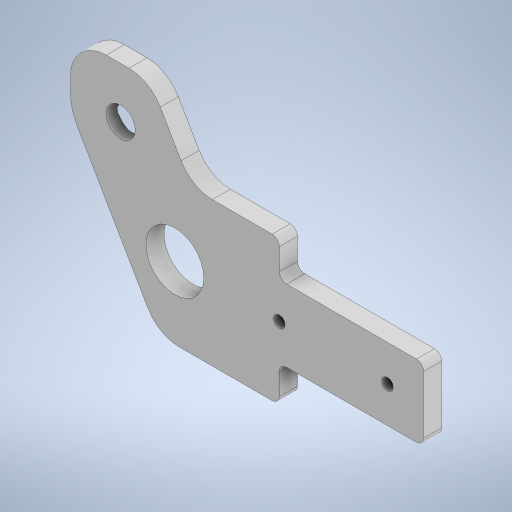
# Autodesk Inventor part: RP_Calf-Link-cover-Inside-Right
Saved by Autodesk Inventor 2024.3 (Build 283343000, 343)
## iProperties
Created: 2025-04-12
Part Number: RP_Calf-Link-cover-Inside-Right
Material: 一般
Document SubType Name: Modeling
Designer: 佐藤智貴
Density: 1 g/cm^3
Appearance: 既定
Author: 佐藤智貴
Autodesk Inventor part; units mm, degrees
ref_plane "YZ Plane" through (0, 0, 0) normal (1, 0, 0) x (0, 1, 0)
ref_plane "XZ Plane" through (0, 0, 0) normal (0, 1, 0) x (-1, 0, 0)
ref_plane "XY Plane" through (0, 0, 0) normal (0, 0, 1) x (1, 0, 0)
sketch "スケッチ1" plane through (0, 0, 0) normal (0, 0, 1) x (1, 0, 0)
  line L0 (0, 0) -> (98, 0)
  line L1 (98, 0) -> (98, 60)
  line L2 (98, 60) -> (0, 60)
  line L3 (0, 60) -> (0, 0)
  line L4 (98, 0) -> (29, 0)
  line L5 (29, 0) -> (29, 40)
  line L6 (29, 40) -> (98, 40)
  line L7 (98, 40) -> (98, 0)
  line L8 (29, 30) -> (98, 30)
  line L9 (98, 30) -> (98, 10)
  line L10 (98, 10) -> (29, 10)
  line L11 (29, 10) -> (29, 30)
  line L12 (98, 20) -> (0, 20)
  line L13 (29, 20) -> (5.906, 60)
  circle A0 centre (29, 20) radius 8.025
  circle A1 centre (14, 45.9808) radius 4.025
  line L14 (58, 40) -> (58, 0)
  line L15 (16.8756, 13) -> (-6.2184, 53)
  line L16 (41.1244, 27) -> (18.0303, 67)
  circle A2 centre (14, 45.9808) radius 14
  line L17 (16.8756, 13) -> (25.3526, -1.6825)
  point P0 (58, 30)
  point P1 (33.6188, 40)
  point P2 (22.0718, 60)
  point P3 (0, 45.9808)
  point P4 (1.8756, 38.9808)
  point P5 (24.3812, 0)
  point P6 (58, 0)
  point P7 (58, 10)
  dimension "d0" = 98
  dimension "d1" = 60
  dimension "d2" = 40
  dimension "d3" = 20
  dimension "d4" = 10
  dimension "d5" = 69
  dimension "d6" = 30
  dimension "d7" = 16.05
  dimension "d8" = 30
  dimension "d9" = 8.05
  dimension "d10" = 40
  dimension "d11" = 28
  constraints: 36 end point, 8 parallel, 8 point on line, 5 perpendicular, 3 centre point, 3 horizontal, 3 tangent, 2 coincident, 2 midpoint
  measures "d0" distance of L1.end L2.end
  measures "d1" distance of L0.end L1.end
  measures "d2" distance between parallel lines of L0 L6
  measures "d3" distance between parallel lines of L10 L8
  measures "d4" distance between parallel lines of L0 L10
  measures "d5" distance of L5.end L6.end
  measures "d6" angle of L13 L11
  measures "d7" diameter of A0
  measures "d8" distance of A0.centre A1.centre
  measures "d9" diameter of A1
  measures "d10" distance between parallel lines of L1 L14
  measures "d11" diameter of A2
extrude "押し出し1" add sketch "スケッチ1" along normal blind 5 contours L5 L10 L14 L0 | L0 L17 L15 L12 A0 L5 | L5 A0 L12 L14 L10 | L14 L12 L1 L10 | L14 L8 L1 L12 | L12 A0 L5 L8 L14 | L15 A2 L13 A0 L12 | L8 L16 L6 L14 | A2 L13 A1 | A0 L13 A2 L16 L6 L5 | L8 L5 L6 L16 | L3 L2 L13 A2 | L13 A1 A2 | L13 L2 L16 A2
sketch "スケッチ2" plane through (0, 0, 5) normal (0, 0, 1) x (1, 0, 0)
  line L0 (98, 10) -> (98, 30) projected
  line L1 (98, 20) -> (47.1161, 20)
  point P0 (0, 0)
  point P1 (88, 20)
  point P2 (58, 20)
  dimension "d14" = 10
  dimension "d15" = 30
  constraints: 2 end point, 2 point on line, 1 horizontal, 1 midpoint
  measures "d14" distance from line of L0 point (88, 20)
  measures "d15" distance of point (88, 20) point (58, 20)
hole "穴1" at (88, 20, 5) at (58, 20, 5) direction (0, 0, -1) diameter 3.2 depth 10
fillet "フィレット1" radius 2 6 edges at (58, 40, 2.5) (58, 30, 2.5) (98, 30, 2.5) (98, 10, 2.5) (58, 0, 2.5) (58, 10, 2.5)
fillet "フィレット2" radius 10 4 edges at (24.3812, 0, 2.5) (0, 60, 2.5) (22.0718, 60, 2.5) (33.6188, 40, 2.5)
sketch "スケッチ5" plane through (0, 0, 0) normal (0, 0, -1) x (-1, 0, 0)
  circle A0 centre (-88, 20) radius 1.6 projected
  circle A1 centre (-88, 20) radius 3
  circle A2 centre (-58, 20) radius 1.6 projected
  circle A3 centre (-58, 20) radius 3
  point P0 (0, 0)
  dimension "d38" = 6
  dimension "d39" = 6
  constraints: 2 centre point, 2 coincident
  measures "d38" diameter of A1
  measures "d39" diameter of A3
extrude "押し出し3" cut sketch "スケッチ5" against normal blind 3 contours A0 | A1 | A2 | A3
sketch "スケッチ6" plane through (0, 0, 0) normal (0, 0, -1) x (-1, 0, 0)
  circle A0 centre (-14, 45.9808) radius 4.025 projected
  circle A1 centre (-14, 45.9808) radius 6.6
  line L0 (-8.4, 49.4736) -> (-8.4, 42.4879)
  arc A2 (-8.4, 47.4736) -> (-8.4, 49.4736) centre (-8.4, 48.4736) ccw
  arc A3 (-8.4, 42.4879) -> (-8.4, 44.4879) centre (-8.4, 43.4879) ccw
  point P0 (0, 0)
  dimension "d42" = 13.2
  dimension "d45" = 5.6
  dimension "d46" = 1
  dimension "d47" = 0
  dimension "d48" = 0
  dimension "d49" = 1
  constraints: 6 point on circle, 3 centre point, 2 end point, 2 point on line, 1 coincident, 1 vertical
  measures "d42" diameter of A1
  measures "d45" distance from line of A1.centre L0
  measures "d46" radius of A2
  measures "d47" distance from line of L0 A2.centre
  measures "d48" distance from line of L0 A3.centre
  measures "d49" radius of A3
extrude "押し出し4" cut sketch "スケッチ6" against normal blind 2 contours L0 A1 | A2 A1 | A1 A2 L0 | L0 A3 A1 | A1 A3
equation "\"d49\" = d46"
